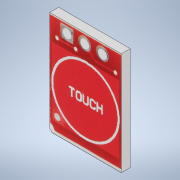
# Autodesk Inventor part: touchsensor
Saved by Autodesk Inventor 2021.2 (Build 252289000, 289)
## iProperties
Created: 2021-10-02
Part Number: touchsensor
Material: Generic
Document SubType Name: Modeling
Designer: Roger
Density: 1 g/cm^3
Appearance: Default
Author: Roger
Autodesk Inventor part; units mm, degrees
ref_plane "YZ Plane" through (0, 0, 0) normal (1, 0, 0) x (0, 1, 0)
ref_plane "XZ Plane" through (0, 0, 0) normal (0, 1, 0) x (-1, 0, 0)
ref_plane "XY Plane" through (0, 0, 0) normal (0, 0, 1) x (1, 0, 0)
sketch "Sketch1" plane through (0, 0, 0) normal (0, 0, 1) x (1, 0, 0)
  line L0 (-4, 5.75) -> (4, 5.75)
  line L1 (4, 5.75) -> (4, -5.75)
  line L2 (4, -5.75) -> (-4, -5.75)
  line L3 (-4, -5.75) -> (-4, 5.75)
  arc A0 (-3.7417, -5.75) -> (-4, -5.4917) centre (-4.2, -5.95) ccw
  point P0 (0, 0)
  point P1 (0, 5.75)
  point P2 (-4, 0)
  dimension "d8" = 8
  dimension "d9" = 11.5
  dimension "d13" = 0.5
  dimension "d14" = 0.2
  dimension "d15" = 0.2
  constraints: 8 end point, 2 midpoint, 2 parallel, 2 point on circle, 2 point on line, 1 centre point, 1 horizontal, 1 horizontal alignment, 1 perpendicular, 1 vertical alignment
  measures "d8" distance of L0.start L0.end
  measures "d9" distance of L0.end L1.end
  measures "d13" radius of A0
  measures "d14" distance from line of L2 A0.centre
  measures "d15" distance from line of A0.centre L3
extrude "Extrusion1" add sketch "Sketch1" along normal blind 1 contours L0 L1 L2 A0 L3
sketch "Sketch2" plane through (0, 0, 1) normal (0, 0, 1) x (1, 0, 0)
  line L0 (4, 5.75) -> (-4, 5.75) projected
  line L1 (-4.1655, 5.7775) -> (4.3538, 5.7775) construction
  line L2 (4.3538, 5.7775) -> (4.3538, -5.6803) construction
  line L3 (4.3538, -5.6803) -> (-4.1655, -5.6803) construction
  line L4 (-4.1655, -5.6803) -> (-4.1655, 5.7775) construction
  point P0 (0, 0)
  constraints: 1 parallel, 2 other
decal "Decal1"
sketch "Sketch3" plane through (0, 0, 0) normal (0, 0, -1) x (-1, 0, 0)
  line L0 (4.2324, 5.7095) -> (4.2324, -5.753) construction
  line L1 (4.2324, -5.753) -> (-4.1099, -5.753) construction
  line L2 (-4.1099, -5.753) -> (-4.1099, 5.7095) construction
  line L3 (-4.1099, 5.7095) -> (4.2324, 5.7095) construction
  line L4 (3.7417, -5.75) -> (-4, -5.75) projected
  point P0 (0, 0)
  constraints: 1 parallel, 2 other
decal "Decal2"
sketch "Sketch4" plane through (0, 0, 0) normal (0, 0, -1) x (-1, 0, 0)
  point P0 (0, 0)
equation "\"d15\" = d14"
body "Solid1"
